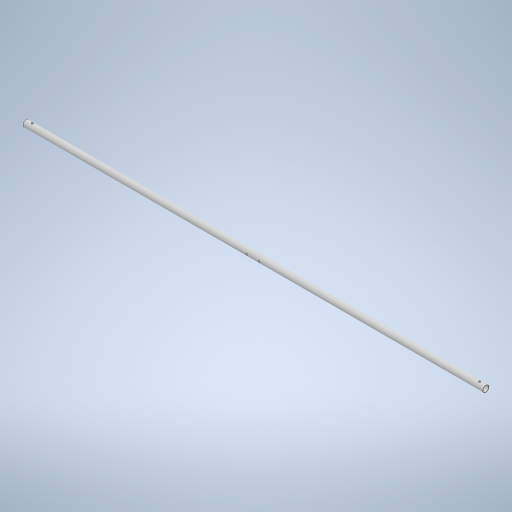
# Autodesk Inventor part: aluminium_pipe_10mm_740mm
Saved by Autodesk Inventor 2024 (Build 280153000, 153)
## iProperties
Created: 2024-09-08
Part Number: aluminium_pipe_10mm_740mm
Material: 일반
Document SubType Name: Modeling
Designer: Gihyeok
Density: 1 g/cm^3
Appearance: 기본값
Author: Gihyeok
Autodesk Inventor part; units mm, degrees
ref_plane "YZ Plane" through (0, 0, 0) normal (1, 0, 0) x (0, 1, 0)
ref_plane "XZ Plane" through (0, 0, 0) normal (0, 1, 0) x (-1, 0, 0)
ref_plane "XY Plane" through (0, 0, 0) normal (0, 0, 1) x (1, 0, 0)
sketch "스케치1" plane through (0, 0, 0) normal (1, 0, 0) x (0, 1, 0)
  circle A0 centre (0, 0) radius 5
  circle A1 centre (0, 0) radius 4.5
  dimension "d0" = 10
  dimension "d1" = 9
  constraints: 2 centre point, 2 coincident
  measures "d0" diameter of A0
  measures "d1" diameter of A1
extrude "돌출1" add sketch "스케치1" along normal blind 740
sketch "스케치2" plane through (0, 0, 0) normal (0, 0, 1) x (1, 0, 0)
  circle A0 centre (360, 0) radius 1.5
  circle A1 centre (380, 0) radius 1.5
  line L0 (0, -5) -> (0, 5) projected
  point P0 (0, 0)
  dimension "d4" = 3
  dimension "d5" = 3
  dimension "d8" = 20
  dimension "d9" = 360
  constraints: 2 centre point
  measures "d4" diameter of A0
  measures "d5" diameter of A1
  measures "d8" distance of A0.centre A1.centre
  measures "d9" distance from line of L0 A0.centre
extrude "돌출2" cut sketch "스케치2" along normal mid plane 740
sketch "스케치3" plane through (0, 0, 0) normal (0, 1, 0) x (-1, 0, 0)
  circle A0 centre (-10, 0) radius 1.5
  line L0 (0, 5) -> (0, -5) projected
  circle A1 centre (-730, 0) radius 1.5
  line L1 (-740, 5) -> (-740, -5) projected
  point P0 (0, 0)
  dimension "d10" = 3
  dimension "d11" = 10
  dimension "d12" = 3
  dimension "d13" = 10
  constraints: 2 centre point
  measures "d10" diameter of A0
  measures "d11" distance from line of L0 A0.centre
  measures "d12" diameter of A1
  measures "d13" distance from line of L1 A1.centre
extrude "돌출3" cut sketch "스케치3" along normal mid plane 740
